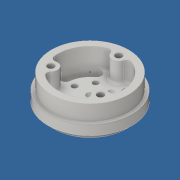
# Autodesk Inventor part: GripperMount_b
Saved by Autodesk Inventor 2016 (Build 200138000, 138)
## iProperties
Created: 2015-09-10
Part Number: GripperMount_b
Material: ABS-Kunststoff
Document SubType Name: Modeling
Designer: 4ndreas
Density: 1.06 g/cm^3
Appearance: Glatt - weiß
Mass: 7.3391 g
Surface Area: 54.5633 cm^2
Volume: 6.92368 cm^3
Author: 4ndreas
Autodesk Inventor part; units mm, degrees
ref_plane "YZ Plane" through (0, 0, 0) normal (1, 0, 0) x (0, 1, 0)
ref_plane "XZ Plane" through (0, 0, 0) normal (0, 1, 0) x (-1, 0, 0)
sketch "Skizze1" plane through (0, 0, 0) normal (0, 0, 1) x (1, 0, 0)
  circle A0 centre (0, 0) radius 17.5
  dimension "d0" = 35
  constraints: 1 centre point, 1 coincident
  measures "d0" diameter of A0
extrude "Extrusion1" add sketch "Skizze1" along normal blind 14
sketch "Skizze2" plane through (0, 0, 0) normal (0, 0, -1) x (-1, 0, 0)
  circle A0 centre (0, 0) radius 9.5
  dimension "d3" = 19
  constraints: 1 centre point, 1 coincident
  measures "d3" diameter of A0
extrude "Extrusion2" cut sketch "Skizze2" against normal blind 2
ref_plane "Arbeitsebene2" through (0, 0, 14) normal (0, 0, 1) x (1, 0, 0)
sketch "Skizze4" plane through (0, 0, 14) normal (0, 0, 1) x (1, 0, 0)
  circle A0 centre (0, 0) radius 9.5 construction
  circle A1 centre (0, 0) radius 17.5 projected
  circle A2 centre (0, 0) radius 14.5
  dimension "d9" = 3
  constraints: 1 centre point, 1 coincident
  measures "d9" radial gap between concentric circles of A2 A1
extrude "Extrusion4" cut sketch "Skizze4" against normal blind 9 contours A2
chamfer "Fase1" distance 1 angle 45 1 edges at (-17.5, 0, 0)
sketch "Skizze5" plane through (0, 0, 5) normal (0, 0, 1) x (1, 0, 0)
  circle A0 centre (0, 0) radius 8.999999
  circle A1 centre (6.822765, 1.565207) radius 0.85
  circle A2 centre (6.691292, -2.055874) radius 0.85
  circle A3 centre (4.766892, -5.126085) radius 0.85
  circle A4 centre (1.565207, -6.822765) radius 0.85
  circle A5 centre (-2.055874, -6.691292) radius 0.85
  circle A6 centre (-5.126085, -4.766892) radius 0.85
  circle A7 centre (-6.822765, -1.565207) radius 0.85
  circle A8 centre (-6.691292, 2.055874) radius 0.85
  circle A9 centre (-4.766892, 5.126085) radius 0.85
  circle A10 centre (-1.565207, 6.822765) radius 0.85
  circle A11 centre (2.055874, 6.691292) radius 0.85
  circle A12 centre (5.126085, 4.766892) radius 0.85
  circle A13 centre (0, 0) radius 4
  line L0 (0, 0) -> (-4.766892, 5.126085) construction
  point P0 (0, 0)
  dimension "d18" = 7
  constraints: 2 end point
  measures "d18" distance of L0.start L0.end
extrude "Extrusion5" [suppressed]
sketch "Skizze6" plane through (0, 0, 14) normal (0, 0, 1) x (1, 0, 0)
  circle A0 centre (0, 0) radius 14.5 projected
  circle A1 centre (0, 0) radius 17.5 projected
sketch "Skizze7" plane through (0, 0, 5) normal (0, 0, 1) x (1, 0, 0)
  circle A0 centre (0, 0) radius 7 construction
  line L0 (3.5, 6.062178) -> (7, 0) construction
  line L1 (7, 0) -> (3.5, -6.062178) construction
  line L2 (3.5, -6.062178) -> (-3.5, -6.062178) construction
  line L3 (-3.5, -6.062178) -> (-7, 0) construction
  line L4 (-7, 0) -> (-3.5, 6.062178) construction
  line L5 (-3.5, 6.062178) -> (3.5, 6.062178) construction
  dimension "d19" = 14
  constraints: 12 end point, 2 coincident, 1 horizontal, 16 other
hole "Bohrung1" at (-3.5, 6.062178, 5) at (-7, 0, 5) at (-3.5, -6.062178, 5) at (3.5, -6.062178, 5) at (7, 0, 5) at (3.5, 6.062178, 5) direction (0, 0, -1) diameter 2.5 end through all
sketch "Skizze8" plane through (0, 0, 14) normal (0, 0, 1) x (1, 0, 0)
  circle A0 centre (0, 13) radius 3
  circle A1 centre (0, 0) radius 14.5
  circle A2 centre (0, 0) radius 17.5
  circle A3 centre (0, 0) radius 14.5
  line L0 (0, 0) -> (0, 13) construction
  line L1 (-3, 13) -> (-3, 14.186261)
  line L2 (3, 13) -> (3, 14.186261)
  dimension "d27" = 6
  dimension "d38" = 13
  constraints: 6 end point, 6 point on circle, 2 parallel, 2 tangent, 1 centre point, 1 vertical
  measures "d27" diameter of A0
  measures "d38" distance of L0.start L0.end
extrude "Extrusion6" add sketch "Skizze8" against normal up to surface (9 mm away) contours A0 A1 | L1 A1 A0 | A0 A1 L2 picked at (0.120537, 12.988009)
fillet "Rundung1" radius 2 2 edges at (-3, 14.1863, 9.5) (3, 14.1863, 9.5)
sketch "Skizze9" plane through (0, 0, 14) normal (0, 0, 1) x (1, 0, 0)
  arc A0 (5.550078, 13.395769) -> (2.87073, 12.128846) centre (4.78455, 11.548077) ccw
  arc A1 (-5.550078, 13.395769) -> (5.550078, 13.395769) centre (0, 0) ccw
  arc A2 (-2.87073, 12.128846) -> (-5.550078, 13.395769) centre (-4.78455, 11.548077) ccw
  arc A3 (-2.87073, 12.128846) -> (2.87073, 12.128846) centre (0, 13) ccw
  circle A4 centre (0, 0) radius 17.5
hole "Bohrung2" at (0, 13, 14) direction (0, 0, -1) diameter 3 end through all
sketch "Skizze10" plane through (0, 0, 0) normal (0, 0, -1) x (-1, 0, 0)
  circle A0 centre (0, 13) radius 1.5
  circle A1 centre (0, 0) radius 9.5
  circle A2 centre (0, 0) radius 16.5
  line L0 (2.886751, 13) -> (1.443376, 10.5)
  line L1 (1.443376, 10.5) -> (-1.443376, 10.5)
  line L2 (-1.443376, 10.5) -> (-2.886751, 13)
  line L3 (-2.886751, 13) -> (-1.443376, 15.5)
  line L4 (-1.443376, 15.5) -> (1.443376, 15.5)
  line L5 (1.443376, 15.5) -> (2.886751, 13)
  dimension "d39" = 5
  constraints: 12 end point, 1 coincident, 1 horizontal, 13 other
  measures "d39" distance between parallel lines of L1 L4
extrude "Extrusion7" cut sketch "Skizze10" against normal blind 5 contours A0 | L0 L1 L2 L3 L4 L5
pattern_circular "Runde Anordnung1" count 3 over 360 about axis through (0, 0, 14) along (0, 0, -1) of "Bohrung2", "Extrusion6", "Rundung1", "Extrusion7"
sketch "Skizze12" plane through (0, 0, 5) normal (0, 0, 1) x (1, 0, 0)
  line L0 (-12.701706, -9) -> (-9.814955, -9)
  line L1 (-9.814955, -9) -> (-8.371579, -6.5)
  line L2 (-8.371579, -6.5) -> (-9.814955, -4)
  line L3 (-9.814955, -4) -> (-12.701706, -4)
  line L4 (-12.701706, -4) -> (-14.145082, -6.5)
  line L5 (-14.145082, -6.5) -> (-12.701706, -9)
  circle A0 centre (-11.25833, -6.5) radius 1.5
  line L6 (14.145082, -6.5) -> (12.701706, -4)
  line L7 (12.701706, -4) -> (9.814955, -4)
  line L8 (9.814955, -4) -> (8.371579, -6.5)
  line L9 (8.371579, -6.5) -> (9.814955, -9)
  line L10 (9.814955, -9) -> (12.701706, -9)
  line L11 (12.701706, -9) -> (14.145082, -6.5)
  circle A1 centre (11.25833, -6.5) radius 1.5
  arc A2 (11.939254, -3.578298) -> (14.376115, -1.891376) centre (12.393203, -1.630497) ccw
  arc A3 (5.550078, 13.395769) -> (2.87073, 12.128846) centre (4.78455, 11.548077) ccw
  arc A4 (-2.87073, 12.128846) -> (2.87073, 12.128846) centre (0, 13) ccw
  arc A5 (-2.87073, 12.128846) -> (-5.550078, 13.395769) centre (-4.78455, 11.548077) ccw
  arc A6 (-5.550078, 13.395769) -> (-14.376115, -1.891376) centre (0, 0) ccw
  arc A7 (-14.376115, -1.891376) -> (-11.939254, -3.578298) centre (-12.393203, -1.630497) ccw
  arc A8 (-9.068524, -8.550548) -> (-11.939254, -3.578298) centre (-11.25833, -6.5) ccw
  arc A9 (-9.068524, -8.550548) -> (-8.826037, -11.504393) centre (-7.608653, -9.91758) ccw
  arc A10 (8.826037, -11.504393) -> (9.068524, -8.550548) centre (7.608653, -9.91758) ccw
  arc A11 (11.939254, -3.578298) -> (9.068524, -8.550548) centre (11.25833, -6.5) ccw
  line L12 (-1.443376, 15.5) -> (-2.886751, 13)
  line L13 (-2.886751, 13) -> (-1.443376, 10.5)
  line L14 (-1.443376, 10.5) -> (1.443376, 10.5)
  line L15 (1.443376, 10.5) -> (2.886751, 13)
  line L16 (2.886751, 13) -> (1.443376, 15.5)
  line L17 (1.443376, 15.5) -> (-1.443376, 15.5)
  circle A12 centre (0, 13) radius 1.5
  circle A13 centre (7, 0) radius 1.25
  circle A14 centre (-3.5, -6.062178) radius 1.25
  circle A15 centre (-3.5, 6.062178) radius 1.25
  circle A16 centre (-7, 0) radius 1.25
  circle A17 centre (3.5, -6.062178) radius 1.25
  circle A18 centre (3.5, 6.062178) radius 1.25
  circle A19 centre (0, 0) radius 17.5
  arc A20 (14.376115, -1.891376) -> (5.550078, 13.395769) centre (0, 0) ccw
  arc A21 (-8.826037, -11.504393) -> (8.826037, -11.504393) centre (0, 0) ccw
  arc A22 (-7.159892, 10.001297) -> (-12.241323, 1.2) centre (0, 0) ccw construction
  arc A23 (-8.440523, 11.790147) -> (-14.430828, 1.414634) centre (0, 0) ccw
  arc A24 (-5.879261, 8.212447) -> (-10.051818, 0.985366) centre (0, 0) ccw
  arc A25 (-5.879261, 8.212447) -> (-8.440523, 11.790147) centre (-7.159892, 10.001297) ccw
  arc A26 (-14.430828, 1.414634) -> (-10.051818, 0.985366) centre (-12.241323, 1.2) ccw
  line L18 (0, 0) -> (-15.155445, 8.75) construction
  line L19 (-3.5, -6.062178) -> (3.5, 6.062178) construction
  point P0 (-14.358773, -2)
  point P1 (-5.447336, 13.435063)
  dimension "d63" = 2.2
  dimension "d64" = 3
  constraints: 12 point on circle, 5 centre point, 5 tangent, 4 end point, 1 coincident, 1 perpendicular, 3 other
  measures "d63" radius of A26
  measures "d64" distance edge to line of A26 L3
extrude "Extrusion8" cut sketch "Skizze12" against normal through all contours A25 A24 A26 A6
pattern_circular "Runde Anordnung2" count 3 over 360 about axis through (0, 0, 0) along (0, 0, 1) of "Extrusion8"
fillet "Rundung3" radius 1 3 edges at (-8.6603, -5, 5) (0, 10, 5) (8.6603, -5, 5)
sketch "Skizze13" plane through (0, 0, 2) normal (0, 0, -1) x (-1, 0, 0)
  circle A0 centre (0, 0) radius 3.5
  dimension "d54" = 7
  constraints: 1 centre point, 1 coincident
  measures "d54" diameter of A0
extrude "Extrusion9" cut sketch "Skizze13" against normal blind 1
sketch "Skizze14" plane through (0, 0, 3) normal (0, 0, -1) x (-1, 0, 0)
  circle A0 centre (0, 0) radius 1.6
  dimension "d57" = 3.2
  constraints: 1 centre point, 1 coincident
  measures "d57" diameter of A0
extrude "Extrusion10" cut sketch "Skizze14" against normal through all
sketch "Skizze15" plane through (-9.814955, -9, 5) normal (0, 0, -1) x (0.5, 0.8660254, 0)
  circle A0 centre (1.443376, -2.5) radius 1.5
  circle A1 centre (12.701706, 17) radius 1.5
  circle A2 centre (12.701706, 17) radius 1.5
  circle A3 centre (23.960036, -2.5) radius 1.5
  circle A4 centre (23.960036, -2.5) radius 1.5
  point P0 (12.701706, 4)
extrude "Extrusion11" add sketch "Skizze15" against normal blind 0.2
sketch "Skizze17" plane through (0, 0, 14) normal (0, 0, 1) x (1, 0, 0)
  point P0 (0, 0)
ref_plane "Arbeitsebene3" through (0, 0, 7) normal (0, 0, 1) x (1, 0, 0)
sketch "Skizze18" plane through (0, 0, 7) normal (0, 0, 1) x (1, 0, 0)
  circle A0 centre (0, 0) radius 19
  circle A1 centre (-11.25833, -6.5) radius 1.5
  circle A2 centre (11.25833, -6.5) radius 1.5
  arc A3 (11.939254, -3.578298) -> (14.376115, -1.891376) centre (12.393203, -1.630497) ccw
  arc A4 (14.376115, -1.891376) -> (5.550078, 13.395769) centre (0, 0) ccw
  arc A5 (5.550078, 13.395769) -> (2.87073, 12.128846) centre (4.78455, 11.548077) ccw
  arc A6 (-2.87073, 12.128846) -> (2.87073, 12.128846) centre (0, 13) ccw
  arc A7 (-2.87073, 12.128846) -> (-5.550078, 13.395769) centre (-4.78455, 11.548077) ccw
  arc A8 (-5.550078, 13.395769) -> (-14.376115, -1.891376) centre (0, 0) ccw
  arc A9 (-14.376115, -1.891376) -> (-11.939254, -3.578298) centre (-12.393203, -1.630497) ccw
  arc A10 (-9.068524, -8.550548) -> (-11.939254, -3.578298) centre (-11.25833, -6.5) ccw
  arc A11 (-9.068524, -8.550548) -> (-8.826037, -11.504393) centre (-7.608653, -9.91758) ccw
  arc A12 (-8.826037, -11.504393) -> (8.826037, -11.504393) centre (0, 0) ccw
  arc A13 (8.826037, -11.504393) -> (9.068524, -8.550548) centre (7.608653, -9.91758) ccw
  arc A14 (11.939254, -3.578298) -> (9.068524, -8.550548) centre (11.25833, -6.5) ccw
  circle A15 centre (0, 13) radius 1.5
  circle A16 centre (0, 0) radius 17.5
  dimension "d66" = 1.5
  dimension "d45" = 40
  constraints: 1 centre point, 1 coincident
  measures "d66" radial gap between concentric circles of A0 A16
extrude "Extrusion12" add sketch "Skizze18" against normal blind 6 contours A0
chamfer "Fase2" distance 1.5 angle 45 1 edges at (-19, 0, 1)
